Autodesk Inventor part; units mm, degrees
(part 4 of 7)
  line L1191 (-73.3785, -52.1517) -> (-73.3854, -53.1021)
  line L1192 (-73.3854, -53.1021) -> (-75.6403, -53.1021)
  line L1193 (-75.6403, -53.1021) -> (-75.6403, -54.7104)
  line L1194 (-75.6403, -54.7104) -> (-73.4082, -54.7104)
  line L1195 (-73.4082, -54.7104) -> (-72.8782, -55.6654)
  line L1196 (-72.8782, -55.6654) -> (-75.6928, -55.6654)
  line L1197 (-56.4611, 24.4344) -> (-57.5218, 25.3515)
  line L1198 (-57.5218, 25.3515) -> (-57.5218, 26.4807)
  line L1199 (-57.5218, 26.4807) -> (-60.7137, 26.4807)
  line L1200 (-60.7137, 26.4807) -> (-61.4611, 27.8123)
  line L1201 (-61.4611, 27.8123) -> (-57.5218, 27.8123)
  line L1202 (-57.5218, 27.8123) -> (-57.5218, 28.9416)
  line L1203 (-57.5218, 28.9416) -> (-56.4611, 29.8554)
  line L1204 (-56.4611, 29.8554) -> (-56.4611, 24.4344)
  line L1205 (-59.7574, 19.1896) -> (-60.743, 20.1263)
  line L1206 (-60.743, 20.1263) -> (-60.743, 23.1746)
  line L1207 (-60.743, 23.1746) -> (-59.7607, 24.108)
  line L1208 (-59.7607, 24.108) -> (-56.4513, 24.108)
  line L1209 (-56.4513, 24.108) -> (-56.4611, 22.7764)
  line L1210 (-56.4611, 22.7764) -> (-59.6823, 22.7764)
  line L1211 (-59.6823, 22.7764) -> (-59.6823, 20.5277)
  line L1212 (-59.6823, 20.5277) -> (-56.4937, 20.5277)
  line L1213 (-56.4937, 20.5277) -> (-55.7365, 19.1896)
  line L1214 (-55.7365, 19.1896) -> (-59.7574, 19.1896)
  line L1215 (-61.4611, 13.4129) -> (-60.7137, 14.7445)
  line L1216 (-60.7137, 14.7445) -> (-59.6889, 14.7445)
  line L1217 (-59.6889, 14.7445) -> (-59.3592, 15.0676)
  line L1218 (-59.3592, 15.0676) -> (-59.3592, 17.2347)
  line L1219 (-59.3592, 17.2347) -> (-60.743, 17.2347)
  line L1220 (-60.743, 17.2347) -> (-60.743, 18.5663)
  line L1221 (-60.743, 18.5663) -> (-56.4611, 18.5663)
  line L1222 (-56.4611, 18.5663) -> (-56.4611, 14.343)
  line L1223 (-56.4611, 14.343) -> (-57.8057, 13.4129)
  line L1224 (-57.8057, 13.4129) -> (-58.762, 14.095)
  line L1225 (-58.762, 14.095) -> (-59.4571, 13.4129)
  line L1226 (-59.4571, 13.4129) -> (-61.4611, 13.4129)
  line L1227 (-57.8873, 14.7771) -> (-57.5218, 15.0578)
  line L1228 (-57.5218, 15.0578) -> (-57.5218, 17.2347)
  line L1229 (-57.5218, 17.2347) -> (-58.2757, 17.2347)
  line L1230 (-58.2757, 17.2347) -> (-58.2757, 15.061)
  line L1231 (-58.2757, 15.061) -> (-57.8873, 14.7771)
  line L1232 (-59.4082, 7.5578) -> (-60.7496, 8.4879)
  line L1233 (-60.7496, 8.4879) -> (-60.7496, 12.7634)
  line L1234 (-60.7496, 12.7634) -> (-56.4611, 12.7634)
  line L1235 (-56.4611, 12.7634) -> (-56.4611, 8.4879)
  line L1236 (-56.4611, 8.4879) -> (-57.8024, 7.5578)
  line L1237 (-57.8024, 7.5578) -> (-58.6053, 8.1191)
  line L1238 (-58.6053, 8.1191) -> (-59.4082, 7.5578)
  line L1239 (-59.4049, 9.0036) -> (-59.0981, 9.2549)
  line L1240 (-59.0981, 9.2549) -> (-59.0981, 11.4318)
  line L1241 (-59.0981, 11.4318) -> (-59.6823, 11.4318)
  line L1242 (-59.6823, 11.4318) -> (-59.6823, 9.2516)
  line L1243 (-59.6823, 9.2516) -> (-59.4049, 9.0036)
  line L1244 (-57.8057, 9.0036) -> (-57.5283, 9.2516)
  line L1245 (-57.5283, 9.2516) -> (-57.5283, 11.4318)
  line L1246 (-57.5283, 11.4318) -> (-58.1125, 11.4318)
  line L1247 (-58.1125, 11.4318) -> (-58.1125, 9.2549)
  line L1248 (-58.1125, 9.2549) -> (-57.8057, 9.0036)
  line L1249 (-59.7574, 1.7484) -> (-60.743, 2.6851)
  line L1250 (-60.743, 2.6851) -> (-60.743, 6.0271)
  line L1251 (-60.743, 6.0271) -> (-59.7607, 6.9605)
  line L1252 (-59.7607, 6.9605) -> (-57.4434, 6.9605)
  line L1253 (-57.4434, 6.9605) -> (-56.4611, 6.0271)
  line L1254 (-56.4611, 6.0271) -> (-56.4611, 2.6851)
  line L1255 (-56.4611, 2.6851) -> (-57.4467, 1.7484)
  line L1256 (-57.4467, 1.7484) -> (-59.7574, 1.7484)
  line L1257 (-59.6823, 3.08) -> (-57.5218, 3.08)
  line L1258 (-57.5218, 3.08) -> (-57.5218, 5.6289)
  line L1259 (-57.5218, 5.6289) -> (-59.6823, 5.6289)
  line L1260 (-59.6823, 5.6289) -> (-59.6823, 3.08)
  line L1261 (2.0619, -0.6586) -> (2.0619, 0.1032)
  line L1262 (2.0619, 0.1032) -> (3.0508, 0.1032)
  line L1263 (3.0508, 0.1032) -> (3.0508, 1.3525)
  line L1264 (3.0508, 1.3525) -> (2.0795, 1.3525)
  line L1265 (2.0795, 1.3525) -> (1.635, 2.1143)
  line L1266 (1.635, 2.1143) -> (4.635, 2.1143)
  line L1267 (4.635, 2.1143) -> (4.635, 1.3525)
  line L1268 (4.635, 1.3525) -> (3.6421, 1.3525)
  line L1269 (3.6421, 1.3525) -> (3.6421, 0.1032)
  line L1270 (3.6421, 0.1032) -> (4.635, 0.1032)
  line L1271 (4.635, 0.1032) -> (4.635, -0.6586)
  line L1272 (4.635, -0.6586) -> (2.0619, -0.6586)
  line L1273 (1.635, -3.8191) -> (2.0795, -3.0535)
  line L1274 (2.0795, -3.0535) -> (2.7786, -3.0535)
  line L1275 (2.7786, -3.0535) -> (2.7786, -1.7806)
  line L1276 (2.7786, -1.7806) -> (2.0619, -1.7806)
  line L1277 (2.0619, -1.7806) -> (2.0658, -1.0189)
  line L1278 (2.0658, -1.0189) -> (4.0514, -1.0189)
  line L1279 (4.0514, -1.0189) -> (4.635, -1.5515)
  line L1280 (4.635, -1.5515) -> (4.635, -3.2865)
  line L1281 (4.635, -3.2865) -> (4.0514, -3.8191)
  line L1282 (4.0514, -3.8191) -> (1.635, -3.8191)
  line L1283 (3.4111, -3.0535) -> (3.9927, -3.0535)
  line L1284 (3.9927, -3.0535) -> (3.9927, -1.7806)
  line L1285 (3.9927, -1.7806) -> (3.4111, -1.7806)
  line L1286 (3.4111, -1.7806) -> (3.4111, -3.0535)
  line L1287 (4.635, -6.9484) -> (3.9927, -6.4275)
  line L1288 (3.9927, -6.4275) -> (3.9927, -4.949)
  line L1289 (3.9927, -4.949) -> (2.7042, -4.949)
  line L1290 (2.7042, -4.949) -> (2.7042, -6.87)
  line L1291 (2.7042, -6.87) -> (2.0619, -6.3452)
  line L1292 (2.0619, -6.3452) -> (2.0619, -4.7179)
  line L1293 (2.0619, -4.7179) -> (2.6454, -4.1873)
  line L1294 (2.6454, -4.1873) -> (4.0416, -4.1873)
  line L1295 (4.0416, -4.1873) -> (4.635, -4.7199)
  line L1296 (4.635, -4.7199) -> (4.635, -6.9484)
  line L1297 (4.635, -9.8015) -> (3.6891, -8.9477)
  line L1298 (3.6891, -8.9477) -> (2.8354, -9.729)
  line L1299 (2.8354, -9.729) -> (2.0795, -9.729)
  line L1300 (2.0795, -9.729) -> (1.635, -8.9673)
  line L1301 (1.635, -8.9673) -> (2.6944, -8.9673)
  line L1302 (2.6944, -8.9673) -> (3.225, -8.5091)
  line L1303 (3.225, -8.5091) -> (2.4946, -7.8354)
  line L1304 (2.4946, -7.8354) -> (2.0619, -7.8354)
  line L1305 (2.0619, -7.8354) -> (2.0658, -7.0737)
  line L1306 (2.0658, -7.0737) -> (4.635, -7.0737)
  line L1307 (4.635, -7.0737) -> (4.635, -7.8354)
  line L1308 (4.635, -7.8354) -> (3.417, -7.8354)
  line L1309 (3.417, -7.8354) -> (4.635, -8.9379)
  line L1310 (4.635, -8.9379) -> (4.635, -9.8015)
  line L1311 (4.635, -12.8563) -> (3.9927, -12.3354)
  line L1312 (3.9927, -12.3354) -> (3.9927, -10.857)
  line L1313 (3.9927, -10.857) -> (2.7042, -10.857)
  line L1314 (2.7042, -10.857) -> (2.7042, -12.778)
  line L1315 (2.7042, -12.778) -> (2.0619, -12.2532)
  line L1316 (2.0619, -12.2532) -> (2.0619, -10.6259)
  line L1317 (2.0619, -10.6259) -> (2.6454, -10.0952)
  line L1318 (2.6454, -10.0952) -> (4.0416, -10.0952)
  line L1319 (4.0416, -10.0952) -> (4.635, -10.6279)
  line L1320 (4.635, -10.6279) -> (4.635, -12.8563)
  line L1321 (2.7042, -15.6644) -> (2.0619, -15.1396)
  line L1322 (2.0619, -15.1396) -> (2.0619, -12.9817)
  line L1323 (2.0619, -12.9817) -> (4.6134, -12.9817)
  line L1324 (4.6134, -12.9817) -> (5.0697, -13.7434)
  line L1325 (5.0697, -13.7434) -> (2.7042, -13.7434)
  line L1326 (2.7042, -13.7434) -> (2.7042, -15.6644)
  line L1327 (2.6572, -18.5097) -> (2.0658, -17.9771)
  line L1328 (2.0658, -17.9771) -> (2.0658, -16.2421)
  line L1329 (2.0658, -16.2421) -> (2.6572, -15.7095)
  line L1330 (2.6572, -15.7095) -> (4.6408, -15.7095)
  line L1331 (4.6408, -15.7095) -> (4.635, -16.4712)
  line L1332 (4.635, -16.4712) -> (2.7022, -16.4712)
  line L1333 (2.7022, -16.4712) -> (2.7022, -17.7441)
  line L1334 (2.7022, -17.7441) -> (4.6134, -17.7441)
  line L1335 (4.6134, -17.7441) -> (5.0697, -18.5097)
  line L1336 (5.0697, -18.5097) -> (2.6572, -18.5097)
  line L1337 (2.8667, -21.8211) -> (2.0619, -21.2924)
  line L1338 (2.0619, -21.2924) -> (2.0619, -18.8583)
  line L1339 (2.0619, -18.8583) -> (4.635, -18.8583)
  line L1340 (4.635, -18.8583) -> (4.635, -21.2924)
  line L1341 (4.635, -21.2924) -> (3.8301, -21.8211)
  line L1342 (3.8301, -21.8211) -> (3.3484, -21.5019)
  line L1343 (3.3484, -21.5019) -> (2.8667, -21.8211)
  line L1344 (2.8686, -20.9947) -> (3.0527, -20.8518)
  line L1345 (3.0527, -20.8518) -> (3.0527, -19.62)
  line L1346 (3.0527, -19.62) -> (2.7042, -19.62)
  line L1347 (2.7042, -19.62) -> (2.7042, -20.8537)
  line L1348 (2.7042, -20.8537) -> (2.8686, -20.9947)
  line L1349 (3.8282, -20.9947) -> (3.9927, -20.8537)
  line L1350 (3.9927, -20.8537) -> (3.9927, -19.62)
  line L1351 (3.9927, -19.62) -> (3.6441, -19.62)
  line L1352 (3.6441, -19.62) -> (3.6441, -20.8518)
  line L1353 (3.6441, -20.8518) -> (3.8282, -20.9947)
  line L1354 (3.2368, -22.7395) -> (3.2368, -22.1559)
  line L1355 (3.2368, -22.1559) -> (3.8791, -22.1559)
  line L1356 (3.8791, -22.1559) -> (3.8791, -22.7395)
  line L1357 (3.8791, -22.7395) -> (3.2368, -22.7395)
  line L1358 (2.0736, -22.7395) -> (2.0736, -22.1559)
  line L1359 (2.0736, -22.1559) -> (2.71, -22.1559)
  line L1360 (2.71, -22.1559) -> (2.71, -22.7395)
  line L1361 (2.71, -22.7395) -> (2.0736, -22.7395)
  line L1362 (4.635, -27.8015) -> (3.9927, -27.2806)
  line L1363 (3.9927, -27.2806) -> (3.9927, -25.8022)
  line L1364 (3.9927, -25.8022) -> (3.6421, -25.8022)
  line L1365 (3.6421, -25.8022) -> (3.6421, -27.4764)
  line L1366 (3.6421, -27.4764) -> (3.0508, -26.9967)
  line L1367 (3.0508, -26.9967) -> (3.0508, -25.8022)
  line L1368 (3.0508, -25.8022) -> (2.0795, -25.8022)
  line L1369 (2.0795, -25.8022) -> (1.635, -25.0404)
  line L1370 (1.635, -25.0404) -> (4.635, -25.0404)
  line L1371 (4.635, -25.0404) -> (4.635, -27.8015)
  line L1372 (2.6572, -30.8857) -> (2.0658, -30.3531)
  line L1373 (2.0658, -30.3531) -> (2.0658, -28.4516)
  line L1374 (2.0658, -28.4516) -> (2.6572, -27.919)
  line L1375 (2.6572, -27.919) -> (4.0436, -27.919)
  line L1376 (4.0436, -27.919) -> (4.635, -28.4516)
  line L1377 (4.635, -28.4516) -> (4.635, -30.3531)
  line L1378 (4.635, -30.3531) -> (4.0436, -30.8857)
  line L1379 (4.0436, -30.8857) -> (2.6572, -30.8857)
  line L1380 (2.7022, -30.124) -> (3.9985, -30.124)
  line L1381 (3.9985, -30.124) -> (3.9985, -28.6807)
  line L1382 (3.9985, -28.6807) -> (2.7022, -28.6807)
  line L1383 (2.7022, -28.6807) -> (2.7022, -30.124)
  line L1384 (1.635, -34.1599) -> (2.0834, -33.3981)
  line L1385 (2.0834, -33.3981) -> (2.6963, -33.3981)
  line L1386 (2.6963, -33.3981) -> (2.8961, -33.216)
  line L1387 (2.8961, -33.216) -> (2.8961, -31.9882)
  line L1388 (2.8961, -31.9882) -> (2.0658, -31.9882)
  line L1389 (2.0658, -31.9882) -> (2.0658, -31.2264)
  line L1390 (2.0658, -31.2264) -> (4.635, -31.2264)
  line L1391 (4.635, -31.2264) -> (4.635, -33.6311)
  line L1392 (4.635, -33.6311) -> (3.8282, -34.1599)
  line L1393 (3.8282, -34.1599) -> (3.2544, -33.7721)
  line L1394 (3.2544, -33.7721) -> (2.8354, -34.1599)
  line L1395 (2.8354, -34.1599) -> (1.635, -34.1599)
  line L1396 (3.7792, -33.3805) -> (3.9985, -33.2199)
  line L1397 (3.9985, -33.2199) -> (3.9985, -31.9882)
  line L1398 (3.9985, -31.9882) -> (3.5462, -31.9882)
  line L1399 (3.5462, -31.9882) -> (3.5462, -33.2199)
  line L1400 (3.5462, -33.2199) -> (3.7792, -33.3805)
  line L1401 (4.635, -37.2852) -> (3.9927, -36.7643)
  line L1402 (3.9927, -36.7643) -> (3.9927, -35.2858)
  line L1403 (3.9927, -35.2858) -> (2.7042, -35.2858)
  line L1404 (2.7042, -35.2858) -> (2.7042, -36.4451)
  line L1405 (2.7042, -36.4451) -> (3.0527, -36.4451)
  line L1406 (3.0527, -36.4451) -> (3.0527, -36.0045)
  line L1407 (3.0527, -36.0045) -> (3.6441, -35.5267)
  line L1408 (3.6441, -35.5267) -> (3.6441, -37.2069)
  line L1409 (3.6441, -37.2069) -> (2.6474, -37.2069)
  line L1410 (2.6474, -37.2069) -> (2.0619, -36.6821)
  line L1411 (2.0619, -36.6821) -> (2.0619, -35.0567)
  line L1412 (2.0619, -35.0567) -> (2.6454, -34.5241)
  line L1413 (2.6454, -34.5241) -> (4.0416, -34.5241)
  line L1414 (4.0416, -34.5241) -> (4.635, -35.0567)
  line L1415 (4.635, -35.0567) -> (4.635, -37.2852)
  line L1416 (4.635, -40.3224) -> (3.9927, -39.8015)
  line L1417 (3.9927, -39.8015) -> (3.9927, -38.323)
  line L1418 (3.9927, -38.323) -> (3.6441, -38.323)
  line L1419 (3.6441, -38.323) -> (3.6441, -39.9973)
  line L1420 (3.6441, -39.9973) -> (3.0527, -39.5176)
  line L1421 (3.0527, -39.5176) -> (3.0527, -38.323)
  line L1422 (3.0527, -38.323) -> (2.7042, -38.323)
  line L1423 (2.7042, -38.323) -> (2.7042, -40.2441)
  line L1424 (2.7042, -40.2441) -> (2.0619, -39.7193)
  line L1425 (2.0619, -39.7193) -> (2.0619, -37.5613)
  line L1426 (2.0619, -37.5613) -> (4.635, -37.5613)
  line L1427 (4.635, -37.5613) -> (4.635, -40.3224)
  line L1428 (-40.0969, -7.1334) -> (-40.0969, -5.8792)
  line L1429 (-40.0969, -5.8792) -> (-39.1511, -5.8792)
  line L1430 (-39.1511, -5.8792) -> (-38.8515, -5.5708)
  line L1431 (-38.8515, -5.5708) -> (-38.8515, -3.5117)
  line L1432 (-38.8515, -3.5117) -> (-40.0705, -3.5117)
  line L1433 (-40.0705, -3.5117) -> (-40.7431, -2.2574)
  line L1434 (-40.7431, -2.2574) -> (-36.2431, -2.2574)
  line L1435 (-36.2431, -2.2574) -> (-36.2431, -6.2522)
  line L1436 (-36.2431, -6.2522) -> (-37.4533, -7.1334)
  line L1437 (-37.4533, -7.1334) -> (-38.3139, -6.4872)
  line L1438 (-38.3139, -6.4872) -> (-38.9396, -7.1334)
  line L1439 (-38.9396, -7.1334) -> (-40.0969, -7.1334)
  line L1440 (-37.5267, -5.8469) -> (-37.1977, -5.5796)
  line L1441 (-37.1977, -5.5796) -> (-37.1977, -3.5117)
  line L1442 (-37.1977, -3.5117) -> (-37.8763, -3.5117)
  line L1443 (-37.8763, -3.5117) -> (-37.8763, -5.5766)
  line L1444 (-37.8763, -5.5766) -> (-37.5267, -5.8469)
  line L1445 (-39.2128, -12.685) -> (-40.0969, -11.8008)
  line L1446 (-40.0969, -11.8008) -> (-40.0969, -8.6373)
  line L1447 (-40.0969, -8.6373) -> (-39.2128, -7.7532)
  line L1448 (-39.2128, -7.7532) -> (-37.1273, -7.7532)
  line L1449 (-37.1273, -7.7532) -> (-36.2431, -8.6373)
  line L1450 (-36.2431, -8.6373) -> (-36.2431, -11.8008)
  line L1451 (-36.2431, -11.8008) -> (-37.1273, -12.685)
  line L1452 (-37.1273, -12.685) -> (-39.2128, -12.685)
  line L1453 (-39.1423, -11.4307) -> (-37.1977, -11.4307)
  line L1454 (-37.1977, -11.4307) -> (-37.1977, -9.0074)
  line L1455 (-37.1977, -9.0074) -> (-39.1423, -9.0074)
  line L1456 (-39.1423, -9.0074) -> (-39.1423, -11.4307)
  line L1457 (-38.8955, -18.1954) -> (-40.1028, -17.3142)
  line L1458 (-40.1028, -17.3142) -> (-40.1028, -13.2695)
  line L1459 (-40.1028, -13.2695) -> (-36.2431, -13.2695)
  line L1460 (-36.2431, -13.2695) -> (-36.2431, -17.3142)
  line L1461 (-36.2431, -17.3142) -> (-37.4504, -18.1954)
  line L1462 (-37.4504, -18.1954) -> (-38.1729, -17.6638)
  line L1463 (-38.1729, -17.6638) -> (-38.8955, -18.1954)
  line L1464 (-37.4533, -16.8325) -> (-37.2036, -16.5946)
  line L1465 (-37.2036, -16.5946) -> (-37.2036, -14.5238)
  line L1466 (-37.2036, -14.5238) -> (-37.7323, -14.5238)
  line L1467 (-37.7323, -14.5238) -> (-37.7323, -16.5916)
  line L1468 (-37.7323, -16.5916) -> (-37.4533, -16.8325)
  line L1469 (-38.8926, -16.8325) -> (-38.6165, -16.5916)
  line L1470 (-38.6165, -16.5916) -> (-38.6165, -14.5238)
  line L1471 (-38.6165, -14.5238) -> (-39.1423, -14.5238)
  line L1472 (-39.1423, -14.5238) -> (-39.1423, -16.5946)
  line L1473 (-39.1423, -16.5946) -> (-38.8926, -16.8325)
  line L1474 (-39.2128, -23.6971) -> (-40.0969, -22.8129)
  line L1475 (-40.0969, -22.8129) -> (-40.0969, -19.6494)
  line L1476 (-40.0969, -19.6494) -> (-39.2128, -18.7653)
  line L1477 (-39.2128, -18.7653) -> (-37.1273, -18.7653)
  line L1478 (-37.1273, -18.7653) -> (-36.2431, -19.6494)
  line L1479 (-36.2431, -19.6494) -> (-36.2431, -22.8129)
  line L1480 (-36.2431, -22.8129) -> (-37.1273, -23.6971)
  line L1481 (-37.1273, -23.6971) -> (-39.2128, -23.6971)
  line L1482 (-39.1423, -22.4428) -> (-37.1977, -22.4428)
  line L1483 (-37.1977, -22.4428) -> (-37.1977, -20.0195)
  line L1484 (-37.1977, -20.0195) -> (-39.1423, -20.0195)
  line L1485 (-39.1423, -20.0195) -> (-39.1423, -22.4428)
  line L1486 (-40.0763, -25.5358) -> (-40.7431, -24.2816)
  line L1487 (-40.7431, -24.2816) -> (-36.2431, -24.2816)
  line L1488 (-36.2431, -24.2816) -> (-36.2431, -25.5358)
  line L1489 (-36.2431, -25.5358) -> (-40.0763, -25.5358)
  line L1490 (-39.1423, -30.5411) -> (-40.1028, -29.6687)
  line L1491 (-40.1028, -29.6687) -> (-40.1028, -26.0851)
  line L1492 (-40.1028, -26.0851) -> (-36.2725, -26.0851)
  line L1493 (-36.2725, -26.0851) -> (-35.591, -27.3394)
  line L1494 (-35.591, -27.3394) -> (-39.1423, -27.3394)
  line L1495 (-39.1423, -27.3394) -> (-39.1423, -30.5411)
  line L1496 (-39.2128, -35.5639) -> (-40.0969, -34.6798)
  line L1497 (-40.0969, -34.6798) -> (-40.0969, -31.5163)
  line L1498 (-40.0969, -31.5163) -> (-39.2128, -30.6321)
  line L1499 (-39.2128, -30.6321) -> (-37.1273, -30.6321)
  line L1500 (-37.1273, -30.6321) -> (-36.2431, -31.5163)
  line L1501 (-36.2431, -31.5163) -> (-36.2431, -34.6798)
  line L1502 (-36.2431, -34.6798) -> (-37.1273, -35.5639)
  line L1503 (-37.1273, -35.5639) -> (-39.2128, -35.5639)
  line L1504 (-39.1423, -34.3097) -> (-37.1977, -34.3097)
  line L1505 (-37.1977, -34.3097) -> (-37.1977, -31.8864)
  line L1506 (-37.1977, -31.8864) -> (-39.1423, -31.8864)
  line L1507 (-39.1423, -31.8864) -> (-39.1423, -34.3097)
  line L1508 (-76.0747, -68.2) -> (-76.0747, -65.2)
  line L1509 (-76.0747, -65.2) -> (-75.5216, -65.2)
  line L1510 (-75.5216, -65.2) -> (-75.098, -66.6726)
  line L1511 (-75.098, -66.6726) -> (-74.6769, -65.2)
  line L1512 (-74.6769, -65.2) -> (-74.1237, -65.2)
  line L1513 (-74.1237, -65.2) -> (-74.1237, -68.2)
  line L1514 (-74.1237, -68.2) -> (-74.6121, -68.2)
  line L1515 (-74.6121, -68.2) -> (-74.6121, -67.5995)
  spline S27 degree 2 poles (-74.6121, -67.5995) (-74.6121, -67.3927) (-74.6021, -66.9766) (-74.5747, -66.563) (-74.5423, -66.1468) (-74.5274, -65.94) knots 0 0 0 1 2 3 4 4 4
  line L1516 (-74.5274, -65.94) -> (-74.9211, -67.298)
  line L1517 (-74.9211, -67.298) -> (-75.2774, -67.298)
  line L1518 (-75.2774, -67.298) -> (-75.6711, -65.94)
  spline S28 degree 2 poles (-75.6711, -65.94) (-75.6561, -66.1468) (-75.6237, -66.563) (-75.5963, -66.9766) (-75.5864, -67.3927) (-75.5864, -67.5995) knots 0 0 0 1 2 3 4 4 4
  line L1519 (-75.5864, -67.5995) -> (-75.5864, -68.2)
  line L1520 (-75.5864, -68.2) -> (-76.0747, -68.2)
  line L1521 (-73.7525, -68.2) -> (-73.0548, -65.2)
  line L1522 (-73.0548, -65.2) -> (-72.4543, -65.2)
  line L1523 (-72.4543, -65.2) -> (-71.7566, -68.2)
  line L1524 (-71.7566, -68.2) -> (-72.2899, -68.2)
  line L1525 (-72.2899, -68.2) -> (-72.4219, -67.5297)
  line L1526 (-72.4219, -67.5297) -> (-73.0872, -67.5297)
  line L1527 (-73.0872, -67.5297) -> (-73.2193, -68.2)
  line L1528 (-73.2193, -68.2) -> (-73.7525, -68.2)
  line L1529 (-72.5016, -67.1385) -> (-72.6835, -66.1992)
  spline S29 degree 2 poles (-72.6835, -66.1992) (-72.7035, -66.1145) (-72.7359, -65.9475) (-72.7533, -65.8603) knots 0 0 0 1 2 2 2
  spline S30 degree 2 poles (-72.7533, -65.8603) (-72.7732, -65.9475) (-72.8056, -66.1145) (-72.8256, -66.1992) knots 0 0 0 1 2 2 2
  line L1530 (-72.8256, -66.1992) -> (-73.0075, -67.1385)
  line L1531 (-73.0075, -67.1385) -> (-72.5016, -67.1385)
  line L1532 (-70.5731, -68.2) -> (-71.3056, -68.2)
  line L1533 (-71.3056, -68.2) -> (-71.3056, -65.2)
  line L1534 (-71.3056, -65.2) -> (-70.5731, -65.2)
  spline S31 degree 2 poles (-70.5731, -65.2) (-70.4286, -65.2) (-70.142, -65.2399) (-69.8804, -65.347) (-69.6636, -65.5214) (-69.5291, -65.7482) (-69.4767, -65.9949) (-69.4767, -66.1219) knots 0 0 0 1 2 3 4 5 6 6 6
  line L1535 (-69.4767, -66.1219) -> (-69.4767, -67.2781)
  spline S32 degree 2 poles (-69.4767, -67.2781) (-69.4767, -67.4051) (-69.5291, -67.6543) (-69.6636, -67.8786) (-69.8804, -68.053) (-70.142, -68.1601) (-70.4286, -68.2) (-70.5731, -68.2) knots 0 0 0 1 2 3 4 5 6 6 6
  line L1536 (-70.7849, -67.8088) -> (-70.5731, -67.8088)
  spline S33 degree 2 poles (-70.5731, -67.8088) (-70.4933, -67.8088) (-70.3339, -67.7789) (-70.1993, -67.7141) (-70.0922, -67.612) (-70.0249, -67.4849) (-69.9975, -67.3478) (-69.9975, -67.2781) knots 0 0 0 1 2 3 4 5 6 6 6
  line L1537 (-69.9975, -67.2781) -> (-69.9975, -66.1219)
  spline S34 degree 2 poles (-69.9975, -66.1219) (-69.9975, -66.0522) (-70.0249, -65.9151) (-70.0922, -65.788) (-70.1993, -65.6859) (-70.3339, -65.6211) (-70.4933, -65.5912) (-70.5731, -65.5912) knots 0 0 0 1 2 3 4 5 6 6 6
  line L1538 (-70.5731, -65.5912) -> (-70.7849, -65.5912)
  line L1539 (-70.7849, -65.5912) -> (-70.7849, -67.8088)
  line L1540 (-68.9236, -68.2) -> (-68.9236, -65.2)
  line L1541 (-68.9236, -65.2) -> (-67.1694, -65.2)
  line L1542 (-67.1694, -65.2) -> (-67.1694, -65.5912)
  line L1543 (-67.1694, -65.5912) -> (-68.4028, -65.5912)
  line L1544 (-68.4028, -65.5912) -> (-68.4028, -66.4458)
  line L1545 (-68.4028, -66.4458) -> (-67.436, -66.4458)
  line L1546 (-67.436, -66.4458) -> (-67.436, -66.837)
  line L1547 (-67.436, -66.837) -> (-68.4028, -66.837)
  line L1548 (-68.4028, -66.837) -> (-68.4028, -67.8088)
  line L1549 (-68.4028, -67.8088) -> (-67.1694, -67.8088)
  line L1550 (-67.1694, -67.8088) -> (-67.1694, -68.2)
  line L1551 (-67.1694, -68.2) -> (-68.9236, -68.2)
  line L1552 (-64.1968, -68.2) -> (-64.1968, -67.8088)
  line L1553 (-64.1968, -67.8088) -> (-63.6387, -67.8088)
  line L1554 (-63.6387, -67.8088) -> (-63.6387, -65.5912)
  line L1555 (-63.6387, -65.5912) -> (-64.1968, -65.5912)
  line L1556 (-64.1968, -65.5912) -> (-64.1968, -65.2)
  line L1557 (-64.1968, -65.2) -> (-62.5548, -65.2)
  line L1558 (-62.5548, -65.2) -> (-62.5548, -65.5912)
  line L1559 (-62.5548, -65.5912) -> (-63.1129, -65.5912)
  line L1560 (-63.1129, -65.5912) -> (-63.1129, -67.8088)
  line L1561 (-63.1129, -67.8088) -> (-62.5548, -67.8088)
  line L1562 (-62.5548, -67.8088) -> (-62.5548, -68.2)
  line L1563 (-62.5548, -68.2) -> (-64.1968, -68.2)
  line L1564 (-61.9269, -68.2) -> (-61.9269, -65.2)
  line L1565 (-61.9269, -65.2) -> (-61.3887, -65.2)
  line L1566 (-61.3887, -65.2) -> (-60.5864, -67.3553)
  spline S35 degree 2 poles (-60.5864, -67.3553) (-60.5988, -67.2357) (-60.6337, -66.999) (-60.6511, -66.7598) (-60.6561, -66.5181) (-60.6561, -66.401) knots 0 0 0 1 2 3 4 4 4
  line L1567 (-60.6561, -66.401) -> (-60.6561, -65.2)
  line L1568 (-60.6561, -65.2) -> (-60.1354, -65.2)
  line L1569 (-60.1354, -65.2) -> (-60.1354, -68.2)
  line L1570 (-60.1354, -68.2) -> (-60.6736, -68.2)
  line L1571 (-60.6736, -68.2) -> (-61.4759, -66.0447)
  spline S36 degree 2 poles (-61.4759, -66.0447) (-61.4634, -66.1643) (-61.4286, -66.401) (-61.4111, -66.6402) (-61.4061, -66.8819) (-61.4061, -66.999) knots 0 0 0 1 2 3 4 4 4
  line L1572 (-61.4061, -66.999) -> (-61.4061, -68.2)
  line L1573 (-61.4061, -68.2) -> (-61.9269, -68.2)
  line L1574 (-56.647, -68.2) -> (-57.1678, -68.2)
  line L1575 (-57.1678, -68.2) -> (-57.1678, -65.2)
  line L1576 (-57.1678, -65.2) -> (-56.3181, -65.2)
  spline S37 degree 2 poles (-56.3181, -65.2) (-56.186, -65.2) (-55.9194, -65.2498) (-55.6902, -65.3669) (-55.5158, -65.5513) (-55.4086, -65.7631) (-55.3712, -65.9949) (-55.3712, -66.1145) knots 0 0 0 1 2 3 4 5 6 6 6
  spline S38 degree 2 poles (-55.3712, -66.1145) (-55.3712, -66.2316) (-55.4086, -66.4658) (-55.5158, -66.6776) (-55.6902, -66.862) (-55.9194, -66.9791) (-56.186, -67.0289) (-56.3181, -67.0289) knots 0 0 0 1 2 3 4 5 6 6 6
  line L1577 (-56.3181, -67.0289) -> (-56.647, -67.0289)
  line L1578 (-56.647, -67.0289) -> (-56.647, -68.2)
  line L1579 (-56.647, -66.6377) -> (-56.3181, -66.6377)
  spline S39 degree 2 poles (-56.3181, -66.6377) (-56.2483, -66.6377) (-56.1163, -66.6003) (-56.0141, -66.5181) (-55.9468, -66.4135) (-55.9045, -66.2939) (-55.892, -66.1767) (-55.892, -66.1145) knots 0 0 0 1 2 3 4 5 6 6 6
  spline S40 degree 2 poles (-55.892, -66.1145) (-55.892, -66.0522) (-55.9045, -65.935) (-55.9468, -65.8154) (-56.0141, -65.7108) (-56.1163, -65.6286) (-56.2483, -65.5912) (-56.3181, -65.5912) knots 0 0 0 1 2 3 4 5 6 6 6
  line L1580 (-56.3181, -65.5912) -> (-56.647, -65.5912)
  line L1581 (-56.647, -65.5912) -> (-56.647, -66.6377)
  spline S41 degree 2 poles (-53.9958, -68.2324) (-54.1279, -68.2324) (-54.387, -68.1875) (-54.6113, -68.0779) (-54.7857, -67.906) (-54.8879, -67.6992) (-54.9302, -67.4774) (-54.9302, -67.3628) knots 0 0 0 1 2 3 4 5 6 6 6
  line L1582 (-54.9302, -67.3628) -> (-54.9302, -66.0372)
  spline S42 degree 2 poles (-54.9302, -66.0372) (-54.9302, -65.9226) (-54.8879, -65.7033) (-54.7857, -65.494) (-54.6113, -65.3221) (-54.387, -65.2125) (-54.1279, -65.1676) (-53.9958, -65.1676) knots 0 0 0 1 2 3 4 5 6 6 6
  spline S43 degree 2 poles (-53.9958, -65.1676) (-53.8663, -65.1676) (-53.6071, -65.2125) (-53.3829, -65.3221) (-53.2085, -65.494) (-53.1063, -65.7033) (-53.0639, -65.9226) (-53.0639, -66.0372) knots 0 0 0 1 2 3 4 5 6 6 6
  line L1583 (-53.0639, -66.0372) -> (-53.0639, -67.3628)
  spline S44 degree 2 poles (-53.0639, -67.3628) (-53.0639, -67.4774) (-53.1063, -67.6992) (-53.2085, -67.906) (-53.3829, -68.0779) (-53.6071, -68.1875) (-53.8663, -68.2324) (-53.9958, -68.2324) knots 0 0 0 1 2 3 4 5 6 6 6
  spline S45 degree 2 poles (-53.9958, -67.8412) (-53.931, -67.8412) (-53.804, -67.8088) (-53.7068, -67.7341) (-53.6395, -67.6369) (-53.5997, -67.5297) (-53.5847, -67.4201) (-53.5847, -67.3628) knots 0 0 0 1 2 3 4 5 6 6 6
  line L1584 (-53.5847, -67.3628) -> (-53.5847, -66.0372)
  spline S46 degree 2 poles (-53.5847, -66.0372) (-53.5847, -65.9799) (-53.5997, -65.8703) (-53.6395, -65.7631) (-53.7068, -65.6659) (-53.804, -65.5912) (-53.931, -65.5588) (-53.9958, -65.5588) knots 0 0 0 1 2 3 4 5 6 6 6
  spline S47 degree 2 poles (-53.9958, -65.5588) (-54.0631, -65.5588) (-54.1902, -65.5912) (-54.2874, -65.6659) (-54.3546, -65.7631) (-54.3945, -65.8703) (-54.4095, -65.9799) (-54.4095, -66.0372) knots 0 0 0 1 2 3 4 5 6 6 6
  line L1585 (-54.4095, -66.0372) -> (-54.4095, -67.3628)
  spline S48 degree 2 poles (-54.4095, -67.3628) (-54.4095, -67.4201) (-54.3945, -67.5297) (-54.3546, -67.6369) (-54.2874, -67.7341) (-54.1902, -67.8088) (-54.0631, -67.8412) (-53.9958, -67.8412) knots 0 0 0 1 2 3 4 5 6 6 6
  line L1586 (-52.4061, -68.2) -> (-52.4061, -65.2)
  line L1587 (-52.4061, -65.2) -> (-51.8879, -65.2)
  line L1588 (-51.8879, -65.2) -> (-51.8879, -67.8088)
  line L1589 (-51.8879, -67.8088) -> (-50.7292, -67.8088)
  line L1590 (-50.7292, -67.8088) -> (-50.7292, -68.2)
  line L1591 (-50.7292, -68.2) -> (-52.4061, -68.2)
  line L1592 (-50.3056, -68.2) -> (-49.608, -65.2)
  line L1593 (-49.608, -65.2) -> (-49.0075, -65.2)
  line L1594 (-49.0075, -65.2) -> (-48.3098, -68.2)
  line L1595 (-48.3098, -68.2) -> (-48.843, -68.2)
  line L1596 (-48.843, -68.2) -> (-48.9751, -67.5297)
  line L1597 (-48.9751, -67.5297) -> (-49.6404, -67.5297)
  line L1598 (-49.6404, -67.5297) -> (-49.7724, -68.2)
  line L1599 (-49.7724, -68.2) -> (-50.3056, -68.2)
  line L1600 (-49.0548, -67.1385) -> (-49.2367, -66.1992)
  spline S49 degree 2 poles (-49.2367, -66.1992) (-49.2566, -66.1145) (-49.289, -65.9475) (-49.3065, -65.8603) knots 0 0 0 1 2 2 2
  spline S50 degree 2 poles (-49.3065, -65.8603) (-49.3264, -65.9475) (-49.3588, -66.1145) (-49.3787, -66.1992) knots 0 0 0 1 2 2 2
  line L1601 (-49.3787, -66.1992) -> (-49.5606, -67.1385)
  line L1602 (-49.5606, -67.1385) -> (-49.0548, -67.1385)
  line L1603 (-47.8588, -68.2) -> (-47.8588, -65.2)
  line L1604 (-47.8588, -65.2) -> (-47.3206, -65.2)
  line L1605 (-47.3206, -65.2) -> (-46.5183, -67.3553)
  spline S51 degree 2 poles (-46.5183, -67.3553) (-46.5307, -67.2357) (-46.5656, -66.999) (-46.583, -66.7598) (-46.588, -66.5181) (-46.588, -66.401) knots 0 0 0 1 2 3 4 4 4
  line L1606 (-46.588, -66.401) -> (-46.588, -65.2)
  line L1607 (-46.588, -65.2) -> (-46.0673, -65.2)
  line L1608 (-46.0673, -65.2) -> (-46.0673, -68.2)
  line L1609 (-46.0673, -68.2) -> (-46.6055, -68.2)
  line L1610 (-46.6055, -68.2) -> (-47.4078, -66.0447)
  spline S52 degree 2 poles (-47.4078, -66.0447) (-47.3953, -66.1643) (-47.3605, -66.401) (-47.343, -66.6402) (-47.338, -66.8819) (-47.338, -66.999) knots 0 0 0 1 2 3 4 4 4
  line L1611 (-47.338, -66.999) -> (-47.338, -68.2)
  line L1612 (-47.338, -68.2) -> (-47.8588, -68.2)
  line L1613 (-44.7815, -68.2) -> (-45.5141, -68.2)
  line L1614 (-45.5141, -68.2) -> (-45.5141, -65.2)
  line L1615 (-45.5141, -65.2) -> (-44.7815, -65.2)
  spline S53 degree 2 poles (-44.7815, -65.2) (-44.637, -65.2) (-44.3505, -65.2399) (-44.0889, -65.347) (-43.8721, -65.5214) (-43.7375, -65.7482) (-43.6852, -65.9949) (-43.6852, -66.1219) knots 0 0 0 1 2 3 4 5 6 6 6
  line L1616 (-43.6852, -66.1219) -> (-43.6852, -67.2781)
  spline S54 degree 2 poles (-43.6852, -67.2781) (-43.6852, -67.4051) (-43.7375, -67.6543) (-43.8721, -67.8786) (-44.0889, -68.053) (-44.3505, -68.1601) (-44.637, -68.2) (-44.7815, -68.2) knots 0 0 0 1 2 3 4 5 6 6 6
  line L1617 (-44.9933, -67.8088) -> (-44.7815, -67.8088)
  spline S55 degree 2 poles (-44.7815, -67.8088) (-44.7018, -67.8088) (-44.5423, -67.7789) (-44.4078, -67.7141) (-44.3006, -67.612) (-44.2334, -67.4849) (-44.206, -67.3478) (-44.206, -67.2781) knots 0 0 0 1 2 3 4 5 6 6 6
  line L1618 (-44.206, -67.2781) -> (-44.206, -66.1219)
  spline S56 degree 2 poles (-44.206, -66.1219) (-44.206, -66.0522) (-44.2334, -65.9151) (-44.3006, -65.788) (-44.4078, -65.6859) (-44.5423, -65.6211) (-44.7018, -65.5912) (-44.7815, -65.5912) knots 0 0 0 1 2 3 4 5 6 6 6
  line L1619 (-44.7815, -65.5912) -> (-44.9933, -65.5912)
  line L1620 (-44.9933, -65.5912) -> (-44.9933, -67.8088)
  point P0 (0, 0)
  point P1 (-13, -51.55)
  point P2 (6.3, -52.6725)
  point P3 (3.25, -48.3)
  point P4 (6.3, -43.9275)
  point P5 (6.3, 5.5275)
  point P6 (3.25, 9.9)
  point P7 (6.3, 14.2725)
  point P8 (-13, 13.15)
  point P9 (-52.4853, 16.5525)
  point P10 (-52.6361, 16.5567)
  point P11 (-52.782, 16.455)
  point P12 (-52.8723, 16.3355)
  point P13 (-52.8771, 16.2639)
  point P14 (-52.8116, 16.2596)
  point P15 (-52.6907, 16.3417)
  point P16 (-52.5799, 16.4236)
  point P17 (-52.5158, 16.4283)
  point P18 (-52.5022, 16.3578)
  point P19 (-52.5431, 16.2141)
  point P20 (-52.5744, 16.0714)
  point P21 (-52.5519, 15.9919)
  point P22 (-52.4934, 15.9917)
  point P23 (-52.4166, 16.0866)
  point P24 (-52.3448, 16.3853)
  point P25 (-52.3892, 16.4903)
  point P26 (-52.2592, 17.7059)
  point P27 (-52.1356, 17.5248)
  point P28 (-51.9251, 17.2559)
  point P29 (-52.0668, 17.0871)
  point P30 (-52.2016, 16.9183)
  point P31 (-52.2433, 17.0666)
  point P32 (-52.2942, 17.1568)
  point P33 (-52.3724, 17.2153)
  point P34 (-52.4441, 17.2262)
  point P35 (-52.4757, 17.1734)
  point P36 (-52.4135, 16.995)
  point P37 (-52.2703, 16.7263)
  point P38 (-52.1124, 16.4814)
  point P39 (-52.0062, 16.3742)
  point P40 (-51.9399, 16.3837)
  point P41 (-51.9205, 16.4197)
  point P42 (-52.0194, 16.6142)
  point P43 (-52.0729, 16.7053)
  point P44 (-52.0849, 16.7705)
  point P45 (-51.9758, 16.9103)
  point P46 (-51.8494, 16.9918)
  point P47 (-51.8138, 16.9861)
  point P48 (-51.7922, 16.9519)
  point P49 (-51.7413, 16.8956)
  point P50 (-51.6638, 16.8676)
  point P51 (-51.5941, 16.8727)
  point P52 (-51.5666, 16.9157)
  point P53 (-51.7978, 17.3259)
  point P54 (-51.9942, 17.6027)
  point P55 (-52.1487, 17.7789)
  point P56 (-52.2663, 17.8528)
  point P57 (-52.2947, 17.8492)
  point P58 (-52.3029, 17.8218)
  point P59 (-50.2693, 16.6848)
  point P60 (-50.9232, 17.2377)
  point P61 (-51.3215, 17.568)
  point P62 (-51.7783, 18.0076)
  point P63 (-53.2491, 19.6107)
  point P64 (-53.5909, 19.9446)
  point P65 (-53.7148, 20.0243)
  point P66 (-53.8118, 20.0504)
  point P67 (-53.9256, 20.0367)
  point P68 (-53.8756, 19.9801)
  point P69 (-53.8193, 19.9314)
  point P70 (-53.7889, 19.8131)
  point P71 (-53.6091, 19.5839)
  point P72 (-53.3854, 19.2823)
  point P73 (-53.3518, 19.1652)
  point P74 (-53.3572, 19.0396)
  point P75 (-53.7947, 15.5136)
  point P76 (-53.8063, 15.279)
  point P77 (-53.3651, 15.3143)
  point P78 (-52.9492, 15.4449)
  point P79 (-52.454, 15.5646)
  point P80 (-51.8054, 15.7225)
  point P81 (-51.1005, 15.9331)
  point P82 (-50.5, 16.1442)
  point P83 (-50.165, 16.3033)
  point P84 (-49.9951, 16.4297)
  point P85 (-51.0336, 16.1022)
  point P86 (-52.5089, 15.7104)
  point P87 (-53.2554, 15.5426)
  point P88 (-53.5973, 15.4916)
  point P89 (-53.5616, 16.0265)
  point P90 (-53.4283, 17.1675)
  point P91 (-53.2683, 18.3468)
  point P92 (-53.1528, 18.9965)
  point P93 (-52.9595, 18.8264)
  point P94 (-52.5133, 18.3589)
  point P95 (-51.707, 17.5381)
  point P96 (-50.763, 16.722)
  point P97 (-50.5151, 16.5069)
  point P98 (-50.4627, 16.4313)
  point P99 (-50.4619, 16.368)
  point P100 (-50.5157, 16.3102)
  point P101 (-50.627, 16.2512)
  point P102 (-52.9213, 20.8512)
  point P103 (-52.0028, 20.7487)
  point P104 (-51.1482, 20.6427)
  point P105 (-50.3026, 20.472)
  point P106 (-49.6145, 20.2728)
  point P107 (-49.376, 20.1738)
  point P108 (-49.2326, 20.0814)
  point P109 (-49.1448, 19.9803)
  point P110 (-49.1099, 19.8939)
  point P111 (-49.1227, 19.7813)
  point P112 (-49.1781, 19.6014)
  point P113 (-49.3806, 18.8791)
  point P114 (-49.4737, 18.2364)
  point P115 (-49.4566, 17.6925)
  point P116 (-49.4065, 17.4636)
  point P117 (-49.3285, 17.2666)
  point P118 (-49.2588, 17.0688)
  point P119 (-49.2499, 16.9453)
  point P120 (-49.1485, 16.652)
  point P121 (-48.8538, 16.0229)
  point P122 (-48.6845, 15.7938)
  point P123 (-48.5307, 15.6547)
  point P124 (-48.2288, 15.6059)
  point P125 (-47.6755, 15.5878)
  point P126 (-47.0347, 15.6011)
  point P127 (-46.4705, 15.6464)
  point P128 (-46.0987, 15.7274)
  point P129 (-45.742, 15.8693)
  point P130 (-45.3942, 16.0747)
  point P131 (-45.0495, 16.3463)
  point P132 (-44.6358, 16.7208)
  point P133 (-44.3421, 17.0243)
  point P134 (-44.1239, 17.307)
  point P135 (-43.9366, 17.6189)
  point P136 (-43.6525, 18.1046)
  point P137 (-43.523, 18.3069)
  point P138 (-43.3617, 18.6996)
  point P139 (-43.2066, 19.1823)
  point P140 (-43.0959, 19.6546)
  point P141 (-43.0398, 20.0564)
  point P142 (-43.0222, 20.4472)
  point P143 (-43.0417, 20.7944)
  point P144 (-43.0973, 21.0657)
  point P145 (-43.3928, 21.709)
  point P146 (-43.7204, 22.2677)
  point P147 (-44.0527, 22.5468)
  point P148 (-44.3747, 22.736)
  point P149 (-45.2196, 23.1839)
  point P150 (-46.252, 23.7057)
  point P151 (-46.6961, 23.8893)
  point P152 (-47.0155, 23.9884)
  point P153 (-47.1564, 24.0454)
  point P154 (-47.7937, 24.3584)
  point P155 (-48.6002, 24.6932)
  point P156 (-49.9175, 25.2277)
  point P157 (-51.3968, 25.8193)
  point P158 (-52.0252, 25.6948)
  point P159 (-51.5813, 25.5448)
  point P160 (-51.358, 25.4849)
  point P161 (-50.9261, 25.3244)
  point P162 (-49.7216, 24.8106)
  point P163 (-48.7354, 24.4045)
  point P164 (-47.862, 24.0482)
  point P165 (-46.8407, 23.6137)
  point P166 (-45.852, 23.1688)
  point P167 (-44.8057, 22.5966)
  point P168 (-44.4801, 22.4154)
  point P169 (-44.2916, 22.3405)
  point P170 (-44.1568, 22.2781)
  point P171 (-43.9901, 22.0986)
  point P172 (-43.7987, 21.8117)
  point P173 (-43.5897, 21.4275)
  point P174 (-43.4509, 21.1367)
  point P175 (-43.3713, 20.9143)
  point P176 (-43.3367, 20.7012)
  point P177 (-43.3327, 20.4387)
  point P178 (-43.3767, 19.7818)
  point P179 (-43.4569, 19.3738)
  point P180 (-43.5854, 18.9863)
  point P181 (-43.7936, 18.5005)
  point P182 (-44.1286, 17.9107)
  point P183 (-44.5098, 17.3449)
  point P184 (-44.8566, 16.9311)
  point P185 (-45.2403, 16.5876)
  point P186 (-45.6158, 16.3115)
  point P187 (-45.9672, 16.1121)
  point P188 (-46.2786, 15.9985)
  point P189 (-46.7506, 15.9386)
  point P190 (-47.4502, 15.8903)
  point P191 (-48.3041, 15.8443)
  point P192 (-48.4868, 16.0355)
  point P193 (-48.6386, 16.2701)
  point P194 (-48.8063, 16.633)
  point P195 (-48.9698, 17.0753)
  point P196 (-49.1671, 17.9451)
  point P197 (-49.1406, 18.3947)
  point P198 (-49.0427, 19.0452)
  point P199 (-48.9463, 19.3465)
  dimension "d87" = 6.5
  dimension "d88" = 6.5
  dimension "d89" = 6.5
  dimension "d90" = 6.5
  dimension "d91" = 6.5
  dimension "d92" = 6.5
  dimension "d93" = 6.5
  dimension "d94" = 6.5
  dimension "d95" = 6.5
  dimension "d96" = 6.5
  dimension "d98" = 5
  dimension "d104" = 6
  dimension "d105" = 32
  dimension "d106" = 5.5
  dimension "d107" = 1
  dimension "d108" = 0
  dimension "d109" = 0
  dimension "d126" = 5
  dimension "d132" = 0
  constraints: 16 end point, 12 coincident, 12 point on line, 11 centre point, 2 point on circle, 15 other
  measures "d87" diameter of A34
  measures "d88" diameter of A35
  measures "d89" diameter of A36
  measures "d90" diameter of A37
  measures "d91" diameter of A39
  measures "d92" diameter of A38
  measures "d93" diameter of A40
  measures "d94" diameter of A41
  measures "d95" diameter of A42
  measures "d96" diameter of A43
  measures "d98" distance between parallel lines of L28 L51
  measures "d104" distance between parallel lines of L51 L55
  measures "d105" distance between parallel lines of L25 L62
  measures "d106" distance between parallel lines of L26 L59
  measures "d107" distance between parallel lines of L33 L65
  measures "d108" distance between parallel lines of L30 L72
  measures "d109" distance between parallel lines of L70 L15
  measures "d126" distance between parallel lines of L27 L83
  measures "d132" distance between parallel lines of L56 L29
extrude "Grawer" cut sketch "Sketch3" against normal blind 0.01 contours L99 L98 L97 L96 L95 L94 L93 L92 L91 L90 L89 L88 L87 L212 L211 L210 L209 L208 L207 L206 L205 L204 L203 L202 L201 L200 L199 L198 L197 L196 L195 L194 L193 L192 L191 L190 L189 L188 L187 L186 L185 L184 L183 L182 L181 L180 L179 L178 L177 L176 L175 L174 L173 L172 L171 L170 L169 L168 L167 L166 L165 L164 L163 L162 L161 L160 L159 L158 L157 L156 L155 L154 L153 L152 L151 L150 L149 L148 L147 L146 L145 L144 L143 L142 L141 L140 L139 L138 L137 L136 L135 L134 L133 L132 L131 L130 L129 L128 L127 L126 L125 L124 L123 L122 L121 L120 L119 L118 L117 L116 L115 L114 L113 L112 L111 L110 L109 L108 L107 L106 L105 L104 L103 L102 L101 L100 A44 L82 | L228 L227 L226 L225 L224 L223 L222 L221 L220 L219 L218 L217 L216 L215 L214 L213 | L256 L255 L254 L253 L252 L251 L250 L249 L248 L247 L246 L245 L244 L243 L242 L241 L240 L239 L238 L237 L236 L235 L234 L233 L232 L231 L230 L229 | L306 L305 L304 L303 L302 L301 L300 L299 L298 L297 L296 L295 L294 L293 L292 L291 L290 L289 L288 L287 L286 L285 L284 L283 L282 L281 L280 L279 L278 L277 L276 L275 L274 | L324 L323 L322 L321 L320 L319 L318 L317 L316 L315 L314 L313 L312 L311 L310 L309 L308 L307 | L325 L326 L327 L328 L329 L330 L331 L332 L333 L334 L335 L336 L337 L338 L339 L340 L341 L342 L343 L344 L345 L346 L347 L348 L349 L350 L351 L352 L353 L354 L355 L356 L357 L358 L359 L360 L361 L362 L363 L364 L365 L366 L367 L368 L369 L370 L371 L372 L373 L374 L375 L376 L377 L378 L379 L380 L381 L382 L383 L384 L385 L386 L387 L388 L389 L390 L391 L392 L393 L394 L395 L396 L397 L398 L399 L400 L401 L402 L403 L404 L405 L406 L407 L408 L409 L410 L411 L412 L413 L414 L415 L416 L417 L418 L419 L420 L421 L422 L423 L424 L425 L426 L427 L428 L429 L430 L431 L432 L433 L434 L435 L436 L437 L438 L439 L440 L441 L442 L443 L444 L445 L446 L447 L448 L449 L450 L451 L452 L453 L454 L455 L456 L457 L458 L459 L460 L461 L462 L463 L464 L465 L466 L467 L468 L469 L470 L471 L472 L473 L474 L475 L476 L477 L478 L479 L480 L481 L482 L483 L484 L485 L486 L487 L488 L489 L490 L491 L492 L493 L494 L495 L496 L497 L498 L499 L500 L501 L502 L503 L504 L505 L506 L507 L508 L509 L510 L511 L512 L513 L514 L515 L516 L517 L518 L519 L520 L521 L522 L523 L524 L525 L526 L527 L528 L529 L530 L531 L532 L533 L534 L535 L536 L537 L538 L539 L540 L541 L542 L543 L544 L545 L546 L547 L548 L549 L550 L551 L552 L553 L554 L555 L556 L557 L558 L559 L560 L561 L562 L563 L564 L565 L566 L567 L568 L569 L570 L571 L572 L573 L574 L575 L576 L577 L578 L579 L580 L581 L582 L583 L584 L585 L586 L587 L588 L589 L590 L591 L592 L593 L594 L595 L596 L597 L598 L599 L600 L601 L602 L603 L604 L605 L606 L607 L608 L609 L610 L611 L612 L613 L614 L615 L616 L617 L618 L619 L620 L621 L622 L623 L624 L625 L626 L627 L628 L629 L630 L631 L632 L633 L634 L635 L636 L637 L638 L639 L640 L641 L642 L643 L644 L645 L646 L647 L648 L649 L650 L651 L652 L653 L654 L655 L656 L657 L658 L659 L660 L661 L662 L663 L664 L665 L666 L667 L668 L669 L670 L671 L672 L673 L674 L675 L676 L677 L678 L679 L680 L681 L682 L683 L684 L685 L686 L687 L688 L689 L690 L691 L692 L693 L694 L695 L696 L697 L698 L699 L700 L701 L702 L703 L704 L705 L706 L707 L708 L709 L710 L711 L712 L713 L714 L715 L716 L717 L718 L719 L720 L721 L722 L723 L724 L725 L726 L727 L728 L729 L730 L731 L732 | L733 L734 L735 L736 L737 L738 L739 L740 L741 L742 L743 L744 L745 L746 L747 L748 L749 L750 L751 L752 L753 L754 L755 L756 L757 L758 L759 L760 L761 L762 L763 L764 L765 L766 L767 L768 L769 L770 L771 L772 L773 L774 L775 L776 L777 L778 L779 L780 L781 L782 L783 L784 L785 | L786 L787 L788 L789 L790 L791 L792 L793 L794 L795 L796 L797 L798 L799 L800 L801 L802 L803 L804 L805 L806 L807 L808 L809 L810 L811 L812 L813 L814 L815 L816 L817 L818 L819 L820 L821 L822 L823 L824 L825 L826 L827 L828 L829 L830 L831 L832 L833 L834 L835 L836 L837 L838 L839 L840 L841 L842 L843 | L844 L845 L846 L847 L848 L849 L850 L851 L852 L853 L854 L855 L856 | L857 L858 L859 L860 L861 L862 L863 L864 L865 L866 L867 L868 L869 L870 L871 L872 L873 L874 L875 L876 L877 L878 L879 L880 L881 L882 L883 L884 L885 L886 | L887 L888 L889 L890 L891 L892 L893 L894 L895 L896 L897 L898 L899 L900 L901 L902 L903 L904 L905 L906 L907 L908 L909 L910 L911 L912 L913 L914 L915 | L916 L917 L918 L919 L920 L921 L922 L923 L924 L925 L926 L927 L928 L929 L930 L931 L932 L933 L934 L935 L936 L937 L938 L939 L940 L941 L942 L943 L944 L945 L946 L947 L948 L949 L950 L951 L952 L953 L954 L955 L956 L957 L958 L959 L960 L961 L962 L963 | L964 L965 L966 L967 L968 L969 L970 L971 L972 L973 L974 L975 L976 L977 L978 L979 L980 | S0 S1 L981 L982 L983 L984 L985 L986 L987 L988 L989 L990 S2 S3 L991 L992 L993 | S4 L994 S5 L995 L996 L997 L998 L999 L1000 L1001 L1002 L1003 S6 L1004 | L1009 L1010 L1011 L1012 L1013 L1014 L1015 L1016 L1017 L1018 L1019 L1020 L1021 L1022 L1023 L1024 | S8 S9 L1025 L1026 S10 S11 S12 L1027 L1028 L1029 L1030 S13 S14 L1031 S15 S16 L1032 L1033 L1034 | L1035 L1036 L1037 L1038 L1039 L1040 L1041 L1042 L1043 L1044 L1045 L1046 L1047 L1048 L1049 L1050 L1051 | L1052 L1053 L1054 L1055 L1056 L1057 L1058 L1059 L1060 | L1061 L1062 L1063 L1064 L1065 L1066 L1067 | S17 S18 L1068 S19 S20 S21 L1069 L1070 L1071 S22 | L1073 L1074 L1075 L1076 L1077 L1078 L1079 L1080 L1081 L1082 L1083 L1084 L1085 L1086 L1087 L1088 | L1089 L1090 L1091 L1092 L1093 L1094 L1095 | L1101 L1102 L1103 L1104 L1105 L1106 | L1107 L1108 L1109 L1110 L1111 L1112 L1113 L1114 L1115 L1116 | L1117 L1118 L1119 L1120 L1121 L1122 L1123 L1124 L1125 L1126 L1127 L1128 L1129 L1130 L1131 L1132 | L1133 L1134 L1135 L1136 L1137 L1138 L1139 L1140 L1141 L1142 | L1143 L1144 L1145 L1146 L1147 L1148 L1149 | L1155 L1156 L1157 L1158 L1159 L1160 | L1161 L1162 L1163 L1164 L1165 L1166 L1167 L1168 L1169 L1170 | L1171 L1172 L1173 L1174 L1175 L1176 L1177 L1178 L1179 L1180 L1181 L1182 L1183 L1184 L1185 L1186 | L1187 L1188 L1189 L1190 L1191 L1192 L1193 L1194 L1195 L1196 | L1197 L1198 L1199 L1200 L1201 L1202 L1203 L1204 | L1205 L1206 L1207 L1208 L1209 L1210 L1211 L1212 L1213 L1214 | L1215 L1216 L1217 L1218 L1219 L1220 L1221 L1222 L1223 L1224 L1225 L1226 | L1232 L1233 L1234 L1235 L1236 L1237 L1238 | L1249 L1250 L1251 L1252 L1253 L1254 L1255 L1256 | L1261 L1262 L1263 L1264 L1265 L1266 L1267 L1268 L1269 L1270 L1271 L1272 | L1273 L1274 L1275 L1276 L1277 L1278 L1279 L1280 L1281 L1282 | L1287 L1288 L1289 L1290 L1291 L1292 L1293 L1294 L1295 L1296 | L1297 L1298 L1299 L1300 L1301 L1302 L1303 L1304 L1305 L1306 L1307 L1308 L1309 L1310 | L1311 L1312 L1313 L1314 L1315 L1316 L1317 L1318 L1319 L1320 | L1321 L1322 L1323 L1324 L1325 L1326 | L1327 L1328 L1329 L1330 L1331 L1332 L1333 L1334 L1335 L1336 | L1337 L1338 L1339 L1340 L1341 L1342 L1343 | L1354 L1355 L1356 L1357 | L1358 L1359 L1360 L1361 | L1362 L1363 L1364 L1365 L1366 L1367 L1368 L1369 L1370 L1371 | L1372 L1373 L1374 L1375 L1376 L1377 L1378 L1379 | L1384 L1385 L1386 L1387 L1388 L1389 L1390 L1391 L1392 L1393 L1394 L1395 | L1401 L1402 L1403 L1404 L1405 L1406 L1407 L1408 L1409 L1410 L1411 L1412 L1413 L1414 L1415 | L1416 L1417 L1418 L1419 L1420 L1421 L1422 L1423 L1424 L1425 L1426 L1427 | L1428 L1429 L1430 L1431 L1432 L1433 L1434 L1435 L1436 L1437 L1438 L1439 | L1445 L1446 L1447 L1448 L1449 L1450 L1451 L1452 | L1457 L1458 L1459 L1460 L1461 L1462 L1463 | L1474 L1475 L1476 L1477 L1478 L1479 L1480 L1481 | L1486 L1487 L1488 L1489 | L1490 L1491 L1492 L1493 L1494 L1495 | L1496 L1497 L1498 L1499 L1500 L1501 L1502 L1503 | L1508 L1509 L1510 L1511 L1512 L1513 L1514 L1515 S27 L1516 L1517 L1518 S28 L1519 L1520 | L1521 L1522 L1523 L1524 L1525 L1526 L1527 L1528 | L1532 L1533 L1534 S31 L1535 S32 | L1540 L1541 L1542 L1543 L1544 L1545 L1546 L1547 L1548 L1549 L1550 L1551 | L1552 L1553 L1554 L1555 L1556 L1557 L1558 L1559 L1560 L1561 L1562 L1563 | L1564 L1565 L1566 S35 L1567 L1568 L1569 L1570 L1571 S36 L1572 L1573 | L1574 L1575 L1576 S37 S38 L1577 L1578 | S41 L1582 S42 S43 L1583 S44 | L1586 L1587 L1588 L1589 L1590 L1591 | L1592 L1593 L1594 L1595 L1596 L1597 L1598 L1599 | L1603 L1604 L1605 S51 L1606 L1607 L1608 L1609 L1610 S52 L1611 L1612 | L1613 L1614 L1615 S53 L1616 S54